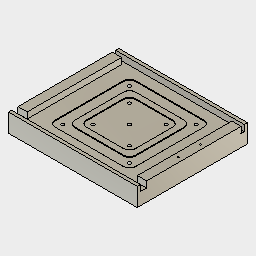
top (Autodesk Fusion 360 design; units mm, degrees)
Autodesk Fusion 360 part; units mm, degrees
note: some values were not read from the file. Chosen so that the rebuilt part matches the saved one: which bodies a step acts on; which face or edge a step refers to. Set by a fixed rule: which sketch regions a step uses.
box "BoxPrimitive1" add length 114.3 width 133.35 height 19.05 placed x (0, 1, 0) y (-1, 0, 0) z (0, 0, 1) at (133.35, 0, 0) makes body 1 in component "Fillet"
fillet "Fillet1" radius 12.7 2 edges at (66.675, 0, 19.05) (66.675, 114.3, 19.05) on bodies 1 in component "Fillet"
box "BoxPrimitive1'" add length 114.3 width 133.35 height 19.05 placed x (0, 1, 0) y (-1, 0, 0) z (0, 0, 1) at (133.35, 0, 0) separate body makes body 2 in component "Inside"
sketch "Sketch2" plane through (0, 0, 19.05) normal (0, 0, 1) x (-1, 0, 0) in component "Inside"
  line L0 (-133.35, -114.3) -> (0, -114.3)
  line L1 (0, -114.3) -> (0, 0)
  line L2 (0, 0) -> (-133.35, 0)
  line L3 (-133.35, 0) -> (-133.35, -114.3)
  line L4 (0, -3.302) -> (-133.35, -3.302)
  line L5 (-133.35, -3.302) -> (-133.35, -9.779)
  line L6 (0, -9.779) -> (0, -3.302)
  line L7 (0, -110.998) -> (-133.35, -110.998)
  line L8 (-133.35, -110.998) -> (-133.35, -107.696)
  line L9 (0, -107.696) -> (0, -110.998)
  line L10 (-123.825, -107.696) -> (-123.825, -9.779)
  line L11 (-9.525, -107.696) -> (-9.525, -9.779)
  line L12 (-133.35, -107.696) -> (-123.825, -107.696)
  line L13 (-9.525, -107.696) -> (0, -107.696)
  line L14 (-133.35, -9.779) -> (-123.825, -9.779)
  line L15 (-9.525, -9.779) -> (0, -9.779)
extrude "Extrude1" cut sketch "Sketch2" against normal blind 6.35 contours L1 L3 L4 L5 L6 L7 L8 L9 L10 L11 L12 L13 L14 L15 bodies 2 in component "Inside"
box "BoxPrimitive1''" add length 50.8 width 50.8 height 0.8128 placed x (0, 1, 0) y (-1, 0, 0) z (0, 0, 1) at (50.8, 0, 0) separate body makes body 3 in component "Copper Touch Pad"
sketch "Sketch2 (2)" plane through (0, 0, 0.8128) normal (0, 0, 1) x (-1, 0, 0) in component "Copper Touch Pad"
  line L0 (-50.8, -50.8) -> (0, -50.8)
  line L1 (0, -50.8) -> (0, 0)
  line L2 (0, 0) -> (-50.8, 0)
  line L3 (-50.8, 0) -> (-50.8, -50.8)
  line L4 (-44.45, 0) -> (-6.35, 0)
  line L5 (0, -6.35) -> (0, -44.45)
  line L6 (-6.35, -50.8) -> (-44.45, -50.8)
  line L7 (-50.8, -44.45) -> (-50.8, -6.35)
  arc A0 (-6.35, -50.8) -> (0, -44.45) centre (-6.35, -44.45) ccw
  arc A1 (-50.8, -44.45) -> (-44.45, -50.8) centre (-44.45, -44.45) ccw
  arc A2 (-44.45, 0) -> (-50.8, -6.35) centre (-44.45, -6.35) ccw
  arc A3 (0, -6.35) -> (-6.35, 0) centre (-6.35, -6.35) ccw
  circle A4 centre (-6.35, -44.45) radius 2.413
  circle A5 centre (-44.45, -44.45) radius 2.413
  circle A6 centre (-6.35, -6.35) radius 2.413
  circle A7 centre (-44.45, -6.35) radius 2.413
  circle A8 centre (-25.4, -25.4) radius 2.413
  point P0 (-25.4, -25.4)
  point P1 (-25.4, -25.4)
  dimension "d116" = 6.35
  dimension "d117" = 4.826
  dimension "d118" = 4.826
  dimension "d119" = 4.826
  dimension "d120" = 4.826
  measures "d116" radius of A0
  measures "d117" diameter of A5
  measures "d118" diameter of A6
  measures "d119" diameter of A7
  measures "d120" diameter of A8
extrude "Extrude1'" cut sketch "Sketch2 (2)" against normal blind 0.8128 contours L0 L3 A1 | L0 L1 A0 | L2 L3 A2 | L1 L2 A3 bodies 3 in component "Copper Touch Pad"
extrude "Extrude2" cut sketch "Sketch2 (2)" against normal blind 0.8128 contours A4 | A5 | A6 | A7 | A8 bodies 3 in component "Copper Touch Pad"
box "BoxPrimitive2" add length 79.4258 width 131.7498 height 19.558 placed x (0, 1, 0) y (-1, 0, 0) z (0, 0, 1) at (131.7498, 0, 0) separate body makes body 4 in component "Touch Test Block"
sketch "Sketch4" plane through (0, 0, 19.558) normal (0, 0, 1) x (-1, 0, 0) in component "Touch Test Block"
  line L0 (-131.7498, -79.4258) -> (0, -79.4258)
  line L1 (0, -79.4258) -> (0, 0)
  line L2 (0, 0) -> (-131.7498, 0)
  line L3 (-131.7498, 0) -> (-131.7498, -79.4258)
  line L4 (-84.9249, -14.3129) -> (-46.8249, -14.3129)
  line L5 (-40.4749, -20.6629) -> (-40.4749, -58.7629)
  line L6 (-46.8249, -65.1129) -> (-84.9249, -65.1129)
  line L7 (-91.2749, -58.7629) -> (-91.2749, -20.6629)
  line L8 (-125.5649, -5.4229) -> (-6.1849, -5.4229)
  line L9 (-6.1849, -5.4229) -> (-6.1849, -74.0029)
  line L10 (-6.1849, -74.0029) -> (-125.5649, -74.0029)
  line L11 (-131.7498, -37.1729) -> (-125.5651, -37.1729)
  line L12 (-125.5651, -42.2529) -> (-131.7498, -42.2529)
  line L13 (-131.7498, -42.2529) -> (-131.7498, -37.1729)
  arc A0 (-46.8249, -65.1129) -> (-40.4749, -58.7629) centre (-46.8249, -58.7629) ccw
  arc A1 (-91.2749, -58.7629) -> (-84.9249, -65.1129) centre (-84.9249, -58.7629) ccw
  arc A2 (-84.9249, -14.3129) -> (-91.2749, -20.6629) centre (-84.9249, -20.6629) ccw
  arc A3 (-40.4749, -20.6629) -> (-46.8249, -14.3129) centre (-46.8249, -20.6629) ccw
  circle A4 centre (-46.8249, -58.7629) radius 1.651
  circle A5 centre (-84.9249, -58.7629) radius 1.651
  circle A6 centre (-65.8749, -39.7129) radius 1.651
  circle A7 centre (-46.8249, -20.6629) radius 1.651
  circle A8 centre (-84.9249, -20.6629) radius 1.651
  line L14 (-125.5649, -74.0029) -> (-125.5651, -42.2529)
  line L15 (-125.5651, -37.1729) -> (-125.5649, -5.4229)
  point P0 (-65.8749, -39.7129)
  point P1 (-65.8749, -39.7129)
  point P2 (-65.8749, -39.7129)
  point P3 (-128.6574, -39.7129)
  point P4 (-128.6574, -39.7129)
  dimension "d149" = 6.35
  measures "d149" radius of A0
extrude "Extrude3" cut sketch "Sketch4" against normal blind 6.35 contours L3 L8 L9 L10 L11 L12 L13 L14 L15 bodies 4 in component "Touch Test Block"
extrude "Extrude4" cut sketch "Sketch4" against normal blind 7.1628 contours L4 L5 L6 L7 A0 A1 A2 A3 bodies 4 in component "Touch Test Block"
extrude "Extrude5" cut sketch "Sketch4" against normal blind 15.875 contours A4 | A5 | A6 | A7 | A8 bodies 4 in component "Touch Test Block"
box "BoxPrimitive1'''" add length 114.3 width 133.35 height 19.05 placed x (0, 1, 0) y (-1, 0, 0) z (0, 0, 1) at (133.35, 0, 0) separate body makes body 5 in component "Inside w/ Touch and Ring"
extrude "Extrude1''" cut sketch "Sketch2" against normal blind 6.35 contours L1 L3 L4 L5 L6 L7 L8 L9 L10 L11 L12 L13 L14 L15 bodies 5 in component "Inside w/ Touch and Ring"
sketch "Sketch2 (3)" plane through (0, 0, 12.7) normal (0, 0, 1) x (-1, 0, 0) in component "Inside w/ Touch and Ring"
  line L0 (-9.525, -107.696) -> (-9.525, -9.779)
  line L1 (-9.525, -9.779) -> (0, -9.779)
  line L2 (0, -9.779) -> (0, -3.302)
  line L3 (0, -3.302) -> (-133.35, -3.302)
  line L4 (-133.35, -3.302) -> (-133.35, -9.779)
  line L5 (-133.35, -9.779) -> (-123.825, -9.779)
  line L6 (-123.825, -9.779) -> (-123.825, -107.696)
  line L7 (-123.825, -107.696) -> (-133.35, -107.696)
  line L8 (-133.35, -107.696) -> (-133.35, -110.998)
  line L9 (-133.35, -110.998) -> (0, -110.998)
  line L10 (0, -110.998) -> (0, -107.696)
  line L11 (0, -107.696) -> (-9.525, -107.696)
  circle A0 centre (-47.625, -77.7875) radius 1.651
  circle A1 centre (-85.725, -77.7875) radius 1.651
  circle A2 centre (-85.725, -39.6875) radius 1.651
  circle A3 centre (-47.625, -39.6875) radius 1.651
  line L12 (-47.498, -33.2105) -> (-85.852, -33.2105)
  line L13 (-92.202, -39.5605) -> (-92.202, -77.9145)
  line L14 (-85.852, -84.2645) -> (-47.498, -84.2645)
  line L15 (-41.148, -77.9145) -> (-41.148, -39.5605)
  arc A4 (-47.498, -84.2645) -> (-41.148, -77.9145) centre (-47.498, -77.9145) ccw
  arc A5 (-92.202, -77.9145) -> (-85.852, -84.2645) centre (-85.852, -77.9145) ccw
  arc A6 (-85.852, -33.2105) -> (-92.202, -39.5605) centre (-85.852, -39.5605) ccw
  arc A7 (-41.148, -39.5605) -> (-47.498, -33.2105) centre (-47.498, -39.5605) ccw
  circle A8 centre (-66.675, -58.7375) radius 1.651
  point P0 (-66.675, -58.7375)
  point P1 (-66.675, -58.7375)
  point P2 (-66.675, -58.7375)
  dimension "d171" = 6.35
  measures "d171" radius of A4
extrude "Extrude2'" cut sketch "Sketch2 (3)" against normal blind 0.8128 contours L12 L13 L14 L15 A4 A5 A6 A7 bodies 5 in component "Inside w/ Touch and Ring"
extrude "Extrude3'" cut sketch "Sketch2 (3)" against normal blind 9.779 contours A0 | A1 | A2 | A3 | A8 bodies 5 in component "Inside w/ Touch and Ring"
box "BoxPrimitive1''''" add length 88.9 width 88.9 height 0.8128 placed x (0, 1, 0) y (-1, 0, 0) z (0, 0, 1) at (88.9, 0, 0) separate body makes body 6 in component "Copper Touch Pad w/ Ring"
sketch "Sketch2 (4)" plane through (0, 0, 0.8128) normal (0, 0, 1) x (-1, 0, 0) in component "Copper Touch Pad w/ Ring"
  line L0 (-88.9, -88.9) -> (0, -88.9)
  line L1 (0, -88.9) -> (0, 0)
  line L2 (0, 0) -> (-88.9, 0)
  line L3 (-88.9, 0) -> (-88.9, -88.9)
  line L4 (-69.85, -12.7) -> (-19.05, -12.7)
  line L5 (-12.7, -19.05) -> (-12.7, -69.85)
  line L6 (-19.05, -76.2) -> (-69.85, -76.2)
  line L7 (-76.2, -69.85) -> (-76.2, -19.05)
  arc A0 (-19.05, -76.2) -> (-12.7, -69.85) centre (-19.05, -69.85) ccw
  arc A1 (-76.2, -69.85) -> (-69.85, -76.2) centre (-69.85, -69.85) ccw
  arc A2 (-69.85, -12.7) -> (-76.2, -19.05) centre (-69.85, -19.05) ccw
  arc A3 (-12.7, -19.05) -> (-19.05, -12.7) centre (-19.05, -19.05) ccw
  point P0 (-44.45, -44.45)
  point P1 (-44.45, -44.45)
  dimension "d183" = 6.35
  dimension "d184" = 6.35
  measures "d183" radius of A0
  measures "d184" radius of A1
extrude "Extrude1'''" cut sketch "Sketch2 (4)" against normal blind 0.8128 contours L4 L5 L6 L7 A0 A1 A2 A3 bodies 6 in component "Copper Touch Pad w/ Ring"
fillet "Fillet1'" radius 6.35 1 edges at (88.9, 0, 0.4064) on bodies 6 in component "Copper Touch Pad w/ Ring"
fillet "Fillet2" radius 6.35 1 edges at (88.9, 88.9, 0.4064) on bodies 6 in component "Copper Touch Pad w/ Ring"
fillet "Fillet3" radius 6.35 1 edges at (0, 88.9, 0.4064) on bodies 6 in component "Copper Touch Pad w/ Ring"
fillet "Fillet4" radius 6.35 1 edges at (0, 0, 0.4064) on bodies 6 in component "Copper Touch Pad w/ Ring"
sketch "Sketch3" plane through (0, 0, 0.8128) normal (0, 0, 1) x (-1, 0, 0) in component "Copper Touch Pad w/ Ring"
  line L0 (-6.35, 0) -> (-82.55, 0)
  circle A0 centre (-81.28, -7.62) radius 2.413
  circle A1 centre (-7.62, -7.62) radius 2.413
  circle A2 centre (-7.62, -81.28) radius 2.413
  circle A3 centre (-81.28, -81.28) radius 2.413
  dimension "d191" = 4.826
  dimension "d192" = 4.826
  dimension "d193" = 4.826
  dimension "d194" = 4.826
  measures "d191" diameter of A0
  measures "d192" diameter of A1
  measures "d193" diameter of A2
  measures "d194" diameter of A3
extrude "Extrude2''" cut sketch "Sketch3" against normal blind 0.8128 bodies 6 in component "Copper Touch Pad w/ Ring"
sketch "Sketch3 (2)" plane through (0, 0, 12.7) normal (0, 0, 1) x (-1, 0, 0) in component "Inside w/ Touch and Ring"
  line L0 (-9.525, -107.696) -> (-9.525, -9.779)
  line L1 (-9.525, -9.779) -> (0, -9.779)
  line L2 (0, -9.779) -> (0, -3.302)
  line L3 (0, -3.302) -> (-133.35, -3.302)
  line L4 (-133.35, -3.302) -> (-133.35, -9.779)
  line L5 (-133.35, -9.779) -> (-123.825, -9.779)
  line L6 (-123.825, -9.779) -> (-123.825, -107.696)
  line L7 (-123.825, -107.696) -> (-133.35, -107.696)
  line L8 (-133.35, -107.696) -> (-133.35, -110.998)
  line L9 (-133.35, -110.998) -> (0, -110.998)
  line L10 (0, -110.998) -> (0, -107.696)
  line L11 (0, -107.696) -> (-9.525, -107.696)
  line L12 (-85.852, -33.2105) -> (-47.498, -33.2105)
  arc A0 (-41.148, -39.5605) -> (-47.498, -33.2105) centre (-47.498, -39.5605) ccw
  line L13 (-41.148, -39.5605) -> (-41.148, -77.9145)
  arc A1 (-47.498, -84.2645) -> (-41.148, -77.9145) centre (-47.498, -77.9145) ccw
  line L14 (-47.498, -84.2645) -> (-85.852, -84.2645)
  arc A2 (-92.202, -77.9145) -> (-85.852, -84.2645) centre (-85.852, -77.9145) ccw
  line L15 (-92.202, -77.9145) -> (-92.202, -39.5605)
  arc A3 (-85.852, -33.2105) -> (-92.202, -39.5605) centre (-85.852, -39.5605) ccw
  line L16 (-97.79, -27.6225) -> (-41.91, -27.6225)
  line L17 (-35.56, -33.9725) -> (-35.56, -89.8525)
  line L18 (-35.56, -89.8525) -> (-97.79, -89.8525)
  line L19 (-97.79, -89.8525) -> (-97.79, -27.6225)
  line L20 (-97.79, -27.6225) -> (-35.56, -89.8525) construction
  line L21 (-35.56, -27.6225) -> (-97.79, -89.8525) construction
  arc A4 (-35.56, -33.9725) -> (-41.91, -27.6225) centre (-41.91, -33.9725) ccw
  line L22 (-106.68, -18.7325) -> (-33.02, -18.7325)
  line L23 (-26.67, -25.0825) -> (-26.67, -98.7425)
  line L24 (-26.67, -98.7425) -> (-106.68, -98.7425)
  line L25 (-106.68, -98.7425) -> (-106.68, -18.7325)
  line L26 (-106.68, -18.7325) -> (-26.67, -98.7425) construction
  arc A5 (-26.67, -25.0825) -> (-33.02, -18.7325) centre (-33.02, -25.0825) ccw
  circle A6 centre (-33.02, -25.0825) radius 1.651
  point P0 (-66.675, -58.7375)
  point P1 (-66.675, -58.7375)
  point P2 (-66.675, -58.7375)
  dimension "d202" = 80.01
  dimension "d204" = 6.35
  measures "d202" distance of L23.end L24.end
  measures "d204" radius of A5
box "BoxPrimitive2'" add length 82.55 width 82.55 height 0.8128 placed x (0, 1, 0) y (-1, 0, 0) z (0, 0, 1) at (82.55, 0, 0) separate body makes body 7 in component "Copper Touch Pad w/ Ring"
sketch "Sketch5" plane through (0, 0, 0.8128) normal (0, 0, 1) x (-1, 0, 0) in component "Copper Touch Pad w/ Ring"
  line L0 (-82.55, -82.55) -> (0, -82.55)
  line L1 (0, -82.55) -> (0, 0)
  line L2 (0, 0) -> (-82.55, 0)
  line L3 (-82.55, 0) -> (-82.55, -82.55)
  line L4 (0, -82.55) -> (-82.55, 0)
  line L5 (0, 0) -> (-82.55, -82.55)
  line L6 (-66.675, -9.525) -> (-15.875, -9.525)
  line L7 (-9.525, -15.875) -> (-9.525, -66.675)
  line L8 (-15.875, -73.025) -> (-66.675, -73.025)
  line L9 (-73.025, -66.675) -> (-73.025, -15.875)
  line L10 (-73.025, -9.525) -> (-9.525, -73.025) construction
  line L11 (-9.525, -9.525) -> (-73.025, -73.025) construction
  arc A0 (-73.025, -66.675) -> (-66.675, -73.025) centre (-66.675, -66.675) ccw
  line L12 (-76.2, 0) -> (-6.35, 0)
  line L13 (0, -6.35) -> (0, -76.2)
  line L14 (-6.35, -82.55) -> (-76.2, -82.55)
  line L15 (-82.55, -76.2) -> (-82.55, -6.35)
  line L16 (-82.55, 0) -> (0, -82.55) construction
  line L17 (0, 0) -> (-82.55, -82.55) construction
  arc A1 (-82.55, -76.2) -> (-76.2, -82.55) centre (-76.2, -76.2) ccw
  line L18 (-71.1651, -71.1651) -> (-75.9247, -75.9247)
  circle A2 centre (-75.9247, -75.9247) radius 2.413
  arc A3 (-6.35, -82.55) -> (0, -76.2) centre (-6.35, -76.2) ccw
  arc A4 (-15.875, -73.025) -> (-9.525, -66.675) centre (-15.875, -66.675) ccw
  line L19 (-11.3849, -71.1651) -> (-6.6253, -75.9247)
  circle A5 centre (-6.6253, -75.9247) radius 2.413
  arc A6 (0, -6.35) -> (-6.35, 0) centre (-6.35, -6.35) ccw
  arc A7 (-9.525, -15.875) -> (-15.875, -9.525) centre (-15.875, -15.875) ccw
  line L20 (-11.3849, -11.3849) -> (-6.6253, -6.6253)
  circle A8 centre (-6.6253, -6.6253) radius 2.413
  arc A9 (-76.2, 0) -> (-82.55, -6.35) centre (-76.2, -6.35) ccw
  arc A10 (-66.675, -9.525) -> (-73.025, -15.875) centre (-66.675, -15.875) ccw
  line L21 (-71.1651, -11.3849) -> (-75.9247, -6.6253)
  circle A11 centre (-75.9247, -6.6253) radius 2.413
  line L22 (-60.325, -15.875) -> (-22.225, -15.875)
  line L23 (-15.875, -22.225) -> (-15.875, -60.325)
  line L24 (-22.225, -66.675) -> (-60.325, -66.675)
  line L25 (-66.675, -60.325) -> (-66.675, -22.225)
  line L26 (-66.675, -15.875) -> (-15.875, -66.675) construction
  line L27 (-15.875, -15.875) -> (-66.675, -66.675) construction
  arc A12 (-22.225, -66.675) -> (-15.875, -60.325) centre (-22.225, -60.325) ccw
  arc A13 (-66.675, -60.325) -> (-60.325, -66.675) centre (-60.325, -60.325) ccw
  arc A14 (-60.325, -15.875) -> (-66.675, -22.225) centre (-60.325, -22.225) ccw
  arc A15 (-15.875, -22.225) -> (-22.225, -15.875) centre (-22.225, -22.225) ccw
  circle A16 centre (-22.225, -60.325) radius 2.413
  circle A17 centre (-60.325, -60.325) radius 2.413
  circle A18 centre (-60.325, -22.225) radius 2.413
  circle A19 centre (-22.225, -22.225) radius 2.413
  circle A20 centre (-41.275, -41.275) radius 2.413
  point P0 (-41.275, -41.275)
  point P1 (-41.275, -41.275)
  point P2 (-80.6901, -80.6901)
  point P3 (-71.1651, -71.1651)
  point P4 (-41.275, -41.275)
  dimension "d213" = 6.35
  dimension "d214" = 4.826
  dimension "d215" = 6.35
  dimension "d216" = 6.35
  dimension "d217" = 6.731
  dimension "d218" = 4.826
  dimension "d219" = 6.35
  dimension "d220" = 6.35
  dimension "d221" = 6.731
  dimension "d222" = 4.826
  dimension "d223" = 6.35
  dimension "d224" = 6.35
  dimension "d225" = 6.731
  dimension "d226" = 4.826
  dimension "d227" = 50.8
  dimension "d228" = 50.8
  dimension "d229" = 6.35
  dimension "d230" = 4.826
  dimension "d231" = 4.826
  dimension "d232" = 4.826
  dimension "d233" = 4.826
  dimension "d234" = 4.826
  measures "d213" radius of A1
  measures "d214" diameter of A2
  measures "d215" radius of A3
  measures "d216" radius of A4
  measures "d217" distance of L19.start L19.end
  measures "d218" diameter of A5
  measures "d219" radius of A6
  measures "d220" radius of A7
  measures "d221" distance of L20.start L20.end
  measures "d222" diameter of A8
  measures "d223" radius of A9
  measures "d224" radius of A10
  measures "d225" distance of L21.start L21.end
  measures "d226" diameter of A11
  measures "d227" distance of A4.centre A0.centre
  measures "d228" distance of A7.centre A4.centre
  measures "d229" radius of A12
  measures "d230" diameter of A16
  measures "d231" diameter of A17
  measures "d232" diameter of A18
  measures "d233" diameter of A19
  measures "d234" diameter of A20
extrude "Extrude3''" cut sketch "Sketch5" against normal blind 0.8128 contours L0 L5 A1 | L3 L5 A1 | L0 L4 A3 | L3 L4 A9 | L5 L18 A2 | L5 L18 A2 | L1 L4 A3 | L2 L4 A9 | L4 L19 A5 | L4 L19 A5 | L4 L21 A11 | L4 L21 A11 | L4 L5 L9 A0 A10 L25 A13 A14 | L4 L5 L8 A0 A4 L24 A12 A13 | L1 L5 A6 | L2 L5 A6 | L4 L5 L7 A4 A7 L23 A12 A15 | L4 L5 L6 A7 A10 L22 A14 A15 | L5 A17 | L5 A17 | L5 L20 A8 | L5 L20 A8 | L4 A16 | L4 A16 | L4 A18 | L4 A18 | L4 L5 A20 | L4 L5 A20 | L4 L5 A20 | L4 L5 A20 | L5 A19 | L5 A19 bodies 7 makes body 8 at (32.8083, 3.175, 0.8128) in component "Copper Touch Pad w/ Ring"
sketch "Sketch4 (2)" plane through (0, 0, 12.7) normal (0, 0, 1) x (-1, 0, 0) in component "Inside w/ Touch and Ring"
  line L0 (-9.525, -107.696) -> (-9.525, -9.779)
  line L1 (-9.525, -9.779) -> (0, -9.779)
  line L2 (0, -9.779) -> (0, -3.302)
  line L3 (0, -3.302) -> (-133.35, -3.302)
  line L4 (-133.35, -3.302) -> (-133.35, -9.779)
  line L5 (-133.35, -9.779) -> (-123.825, -9.779)
  line L6 (-123.825, -9.779) -> (-123.825, -107.696)
  line L7 (-123.825, -107.696) -> (-133.35, -107.696)
  line L8 (-133.35, -107.696) -> (-133.35, -110.998)
  line L9 (-133.35, -110.998) -> (0, -110.998)
  line L10 (0, -110.998) -> (0, -107.696)
  line L11 (0, -107.696) -> (-9.525, -107.696)
  line L12 (-85.852, -33.2105) -> (-47.498, -33.2105)
  arc A0 (-41.148, -39.5605) -> (-47.498, -33.2105) centre (-47.498, -39.5605) ccw
  line L13 (-41.148, -39.5605) -> (-41.148, -77.9145)
  arc A1 (-47.498, -84.2645) -> (-41.148, -77.9145) centre (-47.498, -77.9145) ccw
  line L14 (-47.498, -84.2645) -> (-85.852, -84.2645)
  arc A2 (-92.202, -77.9145) -> (-85.852, -84.2645) centre (-85.852, -77.9145) ccw
  line L15 (-92.202, -77.9145) -> (-92.202, -39.5605)
  arc A3 (-85.852, -33.2105) -> (-92.202, -39.5605) centre (-85.852, -39.5605) ccw
  line L16 (-47.4345, -84.3915) -> (-85.9155, -84.3915)
  line L17 (-91.821, -27.305) -> (-41.529, -27.305)
  line L18 (-101.9492, -17.0498) -> (-31.4008, -17.0498)
  line L19 (-85.9155, -33.0835) -> (-47.4345, -33.0835)
  arc A4 (-101.9492, -17.0498) -> (-108.3627, -23.4633) centre (-101.9492, -23.4632) ccw
  arc A5 (-91.821, -27.305) -> (-98.1075, -33.5915) centre (-91.821, -33.5915) ccw
  line L20 (-41.021, -39.497) -> (-41.021, -77.978)
  line L21 (-24.9872, -23.4633) -> (-24.9872, -94.0118)
  line L22 (-35.2425, -33.5915) -> (-35.2425, -83.8835)
  line L23 (-31.4008, -100.4253) -> (-101.9492, -100.4253)
  line L24 (-108.3628, -94.0118) -> (-108.3628, -23.4633)
  arc A6 (-41.021, -39.497) -> (-47.4345, -33.0835) centre (-47.4345, -39.497) ccw
  arc A7 (-85.9155, -33.0835) -> (-92.329, -39.497) centre (-85.9155, -39.497) ccw
  arc A8 (-92.329, -77.978) -> (-85.9155, -84.3915) centre (-85.9155, -77.978) ccw
  arc A9 (-47.4345, -84.3915) -> (-41.021, -77.978) centre (-47.4345, -77.978) ccw
  line L25 (-41.529, -90.17) -> (-91.821, -90.17)
  arc A10 (-41.529, -90.17) -> (-35.2425, -83.8835) centre (-41.529, -83.8835) ccw
  arc A11 (-31.4008, -100.4253) -> (-24.9872, -94.0118) centre (-31.4007, -94.0118) ccw
  line L26 (-98.1075, -83.8835) -> (-98.1075, -33.5915)
  line L27 (-92.329, -77.978) -> (-92.329, -39.497)
  arc A12 (-98.1075, -83.8835) -> (-91.821, -90.17) centre (-91.821, -83.8835) ccw
  arc A13 (-108.3628, -94.0118) -> (-101.9492, -100.4253) centre (-101.9492, -94.0118) ccw
  arc A14 (-35.2425, -33.5915) -> (-41.529, -27.305) centre (-41.529, -33.5915) ccw
  arc A15 (-24.9872, -23.4633) -> (-31.4008, -17.0498) centre (-31.4007, -23.4633) ccw
  circle A16 centre (-32.0253, -93.3872) radius 1.651
  circle A17 centre (-101.3247, -93.3872) radius 1.651
  circle A18 centre (-32.0253, -24.0878) radius 1.651
  circle A19 centre (-101.3247, -24.0878) radius 1.651
  circle A20 centre (-47.625, -77.7875) radius 1.651
  circle A21 centre (-66.675, -58.7375) radius 1.651
  circle A22 centre (-47.625, -39.6875) radius 1.651
  circle A23 centre (-85.725, -39.6875) radius 1.651
  circle A24 centre (-85.725, -77.7875) radius 1.651
  point P0 (-25.4, -17.4625)
  point P1 (-66.675, -58.7375)
  point P2 (-66.675, -58.7375)
  point P3 (-106.0901, -98.1526)
  point P4 (-96.5651, -88.6276)
  point P5 (-66.675, -58.7375)
  dimension "d269" = 3.302
  measures "d269" diameter of A22
extrude "Extrude4'" add 1 faces at (80.0076, 58.7375, 11.8872) along direction (0, 0, 1) blind 0.8128 on bodies 5 bodies 5 in component "Inside w/ Touch and Ring"
extrude "Extrude5'" add 5 faces at (67.1105, 59.7809, 2.921) (48.2808, 39.8898, 2.921) (48.5864, 78.1325, 2.921) (85.9261, 78.7774, 2.921) (86.1605, 40.7309, 2.921) along direction (0, 0, 1) blind 9.779 on bodies 5 bodies 5 in component "Inside w/ Touch and Ring"
extrude "Extrude6" cut sketch "Sketch4 (2)" against normal blind 9.779 contours A16 | A17 | A18 | A19 | A20 | A21 | A22 | A23 | A24 bodies 5 in component "Inside w/ Touch and Ring"
extrude "Extrude7" cut sketch "Sketch4 (2)" against normal blind 0.8128 contours L12 A0 L13 A1 L14 A2 L15 A3 | L18 A4 L21 L23 L24 A11 A13 A15 bodies 5 in component "Inside w/ Touch and Ring"
move_body "Move1" bodies 8 7 to x (1, 0, 0) y (0, 1, 0) z (0, 0, 1) at (2.54, 2.54, 0) in component "Copper Touch Pad w/ Ring"
sketch "Sketch5 (2)" plane through (0, 0, 19.05) normal (0, 0, 1) x (-1, 0, 0) in component "Inside w/ Touch and Ring"
  line L0 (-133.35, -107.696) -> (-123.825, -107.696)
  line L1 (-123.825, -107.696) -> (-123.825, -9.779)
  line L2 (-123.825, -9.779) -> (-133.35, -9.779)
  line L3 (-133.35, -9.779) -> (-133.35, -107.696)
  line L4 (-128.5875, -58.7375) -> (-128.5875, -70.2361)
  line L5 (-128.5875, -58.7375) -> (-128.5875, -47.2389)
  circle A0 centre (-128.5875, -70.2361) radius 0.8001
  circle A1 centre (-128.5875, -47.2389) radius 0.8001
  point P0 (-128.5875, -58.7375)
  dimension "d276" = 11.4986
  dimension "d277" = 11.4986
  dimension "d278" = 1.6002
  dimension "d279" = 1.6002
  measures "d276" distance of P0 L4.end
  measures "d277" distance of P0 L5.end
  measures "d278" diameter of A0
  measures "d279" diameter of A1
extrude "Extrude8" cut sketch "Sketch5 (2)" against normal blind 4.7625 contours A0 | A1 bodies 5 in component "Inside w/ Touch and Ring"
box "BoxPrimitive1'''''" add length 50.8 width 50.8 height 0.8128 placed x (0, 1, 0) y (-1, 0, 0) z (0, 0, 1) at (50.8, 0, 0) separate body makes body 9 in component "Small Copper Touch Pad w/ Ring"
sketch "Sketch2 (5)" plane through (0, 0, 0.8128) normal (0, 0, 1) x (-1, 0, 0) in component "Small Copper Touch Pad w/ Ring"
  line L0 (-50.8, -50.8) -> (0, -50.8)
  line L1 (0, -50.8) -> (0, 0)
  line L2 (0, 0) -> (-50.8, 0)
  line L3 (-50.8, 0) -> (-50.8, -50.8)
  line L4 (-31.75, -12.7) -> (-19.05, -12.7)
  line L5 (-12.7, -19.05) -> (-12.7, -31.75)
  line L6 (-19.05, -38.1) -> (-31.75, -38.1)
  line L7 (-38.1, -31.75) -> (-38.1, -19.05)
  line L8 (-36.83, -7.62) -> (-13.97, -7.62)
  line L9 (-7.62, -13.97) -> (-7.62, -36.83)
  line L10 (-13.97, -43.18) -> (-36.83, -43.18)
  line L11 (-43.18, -36.83) -> (-43.18, -13.97)
  line L12 (-44.45, 0) -> (-6.35, 0)
  line L13 (0, -6.35) -> (0, -44.45)
  line L14 (-6.35, -50.8) -> (-44.45, -50.8)
  line L15 (-50.8, -44.45) -> (-50.8, -6.35)
  arc A0 (-6.35, -50.8) -> (0, -44.45) centre (-6.35, -44.45) ccw
  arc A1 (-50.8, -44.45) -> (-44.45, -50.8) centre (-44.45, -44.45) ccw
  arc A2 (-44.45, 0) -> (-50.8, -6.35) centre (-44.45, -6.35) ccw
  arc A3 (0, -6.35) -> (-6.35, 0) centre (-6.35, -6.35) ccw
  arc A4 (-7.62, -13.97) -> (-13.97, -7.62) centre (-13.97, -13.97) ccw
  arc A5 (-36.83, -7.62) -> (-43.18, -13.97) centre (-36.83, -13.97) ccw
  arc A6 (-43.18, -36.83) -> (-36.83, -43.18) centre (-36.83, -36.83) ccw
  arc A7 (-13.97, -43.18) -> (-7.62, -36.83) centre (-13.97, -36.83) ccw
  arc A8 (-19.05, -38.1) -> (-12.7, -31.75) centre (-19.05, -31.75) ccw
  arc A9 (-38.1, -31.75) -> (-31.75, -38.1) centre (-31.75, -31.75) ccw
  arc A10 (-31.75, -12.7) -> (-38.1, -19.05) centre (-31.75, -19.05) ccw
  arc A11 (-12.7, -19.05) -> (-19.05, -12.7) centre (-19.05, -19.05) ccw
  circle A12 centre (-45.085, -45.085) radius 2.413
  circle A13 centre (-5.715, -45.085) radius 2.413
  circle A14 centre (-5.715, -5.715) radius 2.413
  circle A15 centre (-45.085, -5.715) radius 2.413
  circle A16 centre (-25.4, -25.4) radius 2.413
  point P0 (-25.4, -25.4)
  point P1 (-25.4, -25.4)
  point P2 (-25.4, -25.4)
  dimension "d289" = 6.35
  dimension "d290" = 4.826
  dimension "d291" = 4.826
  dimension "d292" = 4.826
  dimension "d293" = 4.826
  dimension "d294" = 4.826
  measures "d289" radius of A0
  measures "d290" diameter of A12
  measures "d291" diameter of A13
  measures "d292" diameter of A14
  measures "d293" diameter of A15
  measures "d294" diameter of A16
extrude "Extrude1''''" cut sketch "Sketch2 (5)" against normal blind 0.8128 contours L0 L3 A1 | L0 L1 A0 | L2 L3 A2 | L1 L2 A3 | L8 L9 L10 L11 A4 A5 A6 A7 | A12 | A13 | A14 | A15 | A16 bodies 9 makes body 10 at (25.3399, 16.1312, 0.8128) in component "Small Copper Touch Pad w/ Ring"
box "BoxPrimitive1''''''" add length 114.3 width 133.35 height 19.05 placed x (0, 1, 0) y (-1, 0, 0) z (0, 0, 1) at (133.35, 0, 0) separate body makes body 11 in component "Inside w/ Small Touch"
sketch "Sketch2 (6)" plane through (0, 0, 19.05) normal (0, 0, 1) x (-1, 0, 0) in component "Inside w/ Small Touch"
  line L0 (-133.35, -114.3) -> (0, -114.3)
  line L1 (0, -114.3) -> (0, 0)
  line L2 (0, 0) -> (-133.35, 0)
  line L3 (-133.35, 0) -> (-133.35, -114.3)
  line L4 (0, -3.302) -> (-133.35, -3.302)
  line L5 (-133.35, -3.302) -> (-133.35, -9.779)
  line L6 (0, -9.779) -> (0, -3.302)
  line L7 (0, -110.998) -> (-133.35, -110.998)
  line L8 (-133.35, -110.998) -> (-133.35, -107.696)
  line L9 (0, -107.696) -> (0, -110.998)
  line L10 (-123.825, -107.696) -> (-123.825, -9.779)
  line L11 (-9.525, -107.696) -> (-9.525, -9.779)
  line L12 (-133.35, -107.696) -> (-123.825, -107.696)
  line L13 (-9.525, -107.696) -> (0, -107.696)
  line L14 (-133.35, -9.779) -> (-123.825, -9.779)
  line L15 (-9.525, -9.779) -> (0, -9.779)
extrude "Extrude1'''''" cut sketch "Sketch2 (6)" against normal blind 6.35 contours L1 L3 L4 L5 L6 L7 L8 L9 L10 L11 L12 L13 L14 L15 bodies 11 in component "Inside w/ Small Touch"
sketch "Sketch3 (3)" plane through (0, 0, 12.7) normal (0, 0, 1) x (-1, 0, 0) in component "Inside w/ Small Touch"
  line L0 (-9.525, -107.696) -> (-9.525, -9.779)
  line L1 (-9.525, -9.779) -> (0, -9.779)
  line L2 (0, -9.779) -> (0, -3.302)
  line L3 (0, -3.302) -> (-133.35, -3.302)
  line L4 (-133.35, -3.302) -> (-133.35, -9.779)
  line L5 (-133.35, -9.779) -> (-123.825, -9.779)
  line L6 (-123.825, -9.779) -> (-123.825, -107.696)
  line L7 (-123.825, -107.696) -> (-133.35, -107.696)
  line L8 (-133.35, -107.696) -> (-133.35, -110.998)
  line L9 (-133.35, -110.998) -> (0, -110.998)
  line L10 (0, -110.998) -> (0, -107.696)
  line L11 (0, -107.696) -> (-9.525, -107.696)
  line L12 (-53.7197, -52.2599) -> (-53.7197, -65.0869)
  arc A0 (-60.1332, -71.5004) -> (-53.7197, -65.0869) centre (-60.1332, -65.0869) ccw
  line L13 (-92.2007, -77.9139) -> (-92.2007, -39.4329)
  line L14 (-60.1332, -71.5004) -> (-72.9602, -71.5004)
  arc A1 (-40.8927, -39.4329) -> (-47.3062, -33.0194) centre (-47.3062, -39.4329) ccw
  line L15 (-79.3737, -65.0869) -> (-79.3737, -52.2599)
  line L16 (-48.9471, -47.3589) -> (-48.9471, -69.9903)
  line L17 (-47.3062, -84.3274) -> (-85.7872, -84.3274)
  arc A2 (-72.9602, -45.8464) -> (-79.3737, -52.2599) centre (-72.9602, -52.2599) ccw
  arc A3 (-55.2336, -76.2768) -> (-48.9471, -69.9903) centre (-55.2336, -69.9903) ccw
  line L18 (-72.9602, -45.8464) -> (-60.1332, -45.8464)
  arc A4 (-47.3062, -84.3274) -> (-40.8927, -77.9139) centre (-47.3062, -77.9139) ccw
  arc A5 (-92.2007, -77.9139) -> (-85.7872, -84.3274) centre (-85.7872, -77.9139) ccw
  arc A6 (-84.1515, -69.9903) -> (-77.865, -76.2768) centre (-77.865, -69.9903) ccw
  line L19 (-84.1515, -69.9903) -> (-84.1515, -47.3589)
  arc A7 (-48.9471, -47.3589) -> (-55.2336, -41.0724) centre (-55.2336, -47.3589) ccw
  arc A8 (-53.7197, -52.2599) -> (-60.1332, -45.8464) centre (-60.1332, -52.2599) ccw
  arc A9 (-77.865, -41.0724) -> (-84.1515, -47.3589) centre (-77.865, -47.3589) ccw
  line L20 (-85.7872, -33.0194) -> (-47.3062, -33.0194)
  line L21 (-77.865, -41.0724) -> (-55.2336, -41.0724)
  line L22 (-55.2336, -76.2768) -> (-77.865, -76.2768)
  arc A10 (-79.3737, -65.0869) -> (-72.9602, -71.5004) centre (-72.9602, -65.0869) ccw
  arc A11 (-85.7872, -33.0194) -> (-92.2007, -39.4329) centre (-85.7872, -39.4329) ccw
  line L23 (-40.8927, -39.4329) -> (-40.8927, -77.9139)
  circle A12 centre (-46.863, -78.359) radius 1.651
  circle A13 centre (-86.233, -78.359) radius 1.651
  circle A14 centre (-66.675, -58.7375) radius 1.651
  circle A15 centre (-46.863, -38.989) radius 1.651
  circle A16 centre (-86.233, -38.989) radius 1.651
  point P0 (-66.675, -58.7375)
  point P1 (-66.675, -58.7375)
  point P2 (-66.675, -58.7375)
  point P3 (-66.675, -58.7375)
  point P4 (-41.148, -33.274)
  dimension "d303" = 3.302
  dimension "d304" = 3.302
  dimension "d305" = 3.302
  dimension "d306" = 3.302
  dimension "d307" = 3.302
  measures "d303" diameter of A12
  measures "d304" diameter of A13
  measures "d305" diameter of A14
  measures "d306" diameter of A15
  measures "d307" diameter of A16
extrude "Extrude2'''" cut sketch "Sketch3 (3)" against normal blind 9.525 contours A12 | A13 | A14 | A15 | A16 bodies 11 in component "Inside w/ Small Touch"
extrude "Extrude3'''" cut sketch "Sketch3 (3)" against normal blind 0.8128 contours L12 A0 L14 L15 A2 L18 A8 A10 | L13 A1 L17 A4 A5 L20 A11 L23 bodies 11 in component "Inside w/ Small Touch"
sketch "Sketch4 (3)" plane through (0, 0, 19.05) normal (0, 0, 1) x (-1, 0, 0) in component "Inside w/ Small Touch"
  line L0 (-133.35, -107.696) -> (-123.825, -107.696)
  line L1 (-123.825, -107.696) -> (-123.825, -9.779)
  line L2 (-123.825, -9.779) -> (-133.35, -9.779)
  line L3 (-133.35, -9.779) -> (-133.35, -107.696)
  line L4 (-133.35, -9.779) -> (-133.35, -107.696)
  line L5 (-133.35, -9.779) -> (-133.35, -107.696)
  line L6 (-133.35, -107.696) -> (-123.825, -107.696)
  line L7 (-123.825, -9.779) -> (-133.35, -9.779)
  line L8 (-123.825, -9.779) -> (-133.35, -9.779)
  line L9 (-123.825, -107.696) -> (-123.825, -9.779)
  line L10 (-133.35, -107.696) -> (-123.825, -107.696)
  line L11 (-123.825, -107.696) -> (-123.825, -9.779)
  circle A0 centre (-128.5875, -70.2361) radius 0.8001
  circle A1 centre (-128.5875, -47.2389) radius 0.8001
  circle A2 centre (-128.5875, -70.2361) radius 0.8001
  circle A3 centre (-128.5875, -47.2389) radius 0.8001
  line L12 (-128.5875, -58.7375) -> (-128.5875, -70.2361)
  line L13 (-128.5875, -58.7375) -> (-128.5875, -70.2361)
  line L14 (-128.5875, -58.7375) -> (-128.5875, -47.2389)
  line L15 (-128.5875, -58.7375) -> (-128.5875, -47.2389)
  point P0 (-128.5875, -58.7375)
  dimension "d312" = 11.4986
  dimension "d313" = 11.4986
  dimension "d314" = 1.6002
  dimension "d315" = 1.6002
  measures "d312" distance of P0 A0.centre
  measures "d313" distance of P0 A1.centre
  measures "d314" diameter of A0
  measures "d315" diameter of A1
extrude "Extrude4''" cut sketch "Sketch4 (3)" against normal blind 4.7625 contours A0 A2 | A1 A3 bodies 11 in component "Inside w/ Small Touch"
box "BoxPrimitive1'''''''" add length 76.2 width 76.2 height 0.8128 placed x (0, 1, 0) y (-1, 0, 0) z (0, 0, 1) at (76.2, 0, 0) separate body makes body 12 in component "Circular Touch"
sketch "Sketch2 (7)" plane through (0, 0, 0.8128) normal (0, 0, 1) x (-1, 0, 0) in component "Circular Touch"
  line L0 (-76.2, -76.2) -> (0, -76.2)
  line L1 (0, -76.2) -> (0, 0)
  line L2 (0, 0) -> (-76.2, 0)
  line L3 (-76.2, 0) -> (-76.2, -76.2)
  circle A0 centre (-38.1, -38.1) radius 38.1
  circle A1 centre (-38.1, -38.1) radius 25.4
  circle A2 centre (-38.1, -38.1) radius 29.21
  circle A3 centre (-71.755, -38.1) radius 2.413
  circle A4 centre (-38.1, -71.755) radius 2.413
  circle A5 centre (-4.445, -38.1) radius 2.413
  circle A6 centre (-38.1, -4.445) radius 2.413
  circle A7 centre (-38.1, -38.1) radius 2.413
  point P0 (-38.1, -38.1)
extrude "Extrude1''''''" cut sketch "Sketch2 (7)" against normal blind 0.8128 contours L0 L3 A0 | L0 L1 A0 | L2 L3 A0 | L1 L2 A0 | A2 | A3 | A4 | A5 | A6 | A7 bodies 12 makes body 13 at (20.4659, 39.4818, 0.8128) in component "Circular Touch"
box "BoxPrimitive1''''''''" add length 50.8 width 50.8 height 0.8128 placed x (0, 1, 0) y (-1, 0, 0) z (0, 0, 1) at (50.8, 0, 0) separate body makes body 14 in component "Small Circular Touch"
sketch "Sketch2 (8)" plane through (0, 0, 0.8128) normal (0, 0, 1) x (-1, 0, 0) in component "Small Circular Touch"
  line L0 (-50.8, -50.8) -> (0, -50.8)
  line L1 (0, -50.8) -> (0, 0)
  line L2 (0, 0) -> (-50.8, 0)
  line L3 (-50.8, 0) -> (-50.8, -50.8)
  circle A0 centre (-25.4, -25.4) radius 25.4
  circle A1 centre (-25.4, -25.4) radius 17.78
  circle A2 centre (-46.99, -25.4) radius 2.413
  circle A3 centre (-3.81, -25.4) radius 2.413
  circle A4 centre (-25.4, -25.4) radius 16.129
  circle A5 centre (-25.4, -25.4) radius 2.413
  point P0 (-25.4, -25.4)
extrude "Extrude1'''''''" cut sketch "Sketch2 (8)" against normal blind 0.8128 contours L0 L3 A0 | L0 L1 A0 | L2 L3 A0 | L1 L2 A0 | A1 | A2 | A3 | A5 bodies 14 makes body 15 at (13.912, 26.3212, 0.8128) in component "Small Circular Touch"
extrude "Extrude9" add 1 faces at (32.4911, 93.5494, 2.921) along direction (0, 0, 1) blind 3.175 on bodies 5 bodies 5 in component "Inside w/ Touch and Ring"
extrude "Extrude10" add 1 faces at (32.4911, 93.5494, 6.096) along direction (0, 0, 1) blind 0.254 on bodies 5 bodies 5 in component "Inside w/ Touch and Ring"
extrude "Extrude11" add 1 faces at (48.2733, 78.1618, 2.921) along direction (0, 0, 1) blind 3.429 on bodies 5 bodies 5 in component "Inside w/ Touch and Ring"
extrude "Extrude12" add 5 faces at (31.5324, 23.3215, 2.921) (48.2808, 39.8898, 2.921) (67.1105, 59.7809, 2.921) (86.0681, 78.6953, 2.921) (101.6678, 94.295, 2.921) along direction (0, 0, 1) blind 3.429 on bodies 5 bodies 5 in component "Inside w/ Touch and Ring"
extrude "Extrude13" add 2 faces at (86.1605, 40.7309, 2.921) (101.6678, 24.9957, 2.921) along direction (0, 0, 1) blind 3.429 on bodies 5 bodies 5 in component "Inside w/ Touch and Ring"
extrude "Extrude5''" add 5 faces at (47.5113, 78.7333, 3.175) (86.4341, 79.3489, 3.175) (67.1105, 59.7809, 3.175) (47.5188, 39.1913, 3.175) (86.6685, 40.0324, 3.175) along direction (0, 0, 1) blind 3.429 on bodies 11 bodies 11 in component "Inside w/ Small Touch"
extrude "Extrude6'" cut 5 faces at (47.5113, 78.7333, 6.604) (86.4341, 79.3489, 6.604) (67.1105, 59.7809, 6.604) (47.5188, 39.1913, 6.604) (86.6685, 40.0324, 6.604) along direction (0, 0, -1) blind 0.254 on bodies 11 bodies 11 in component "Inside w/ Small Touch"
box "BoxPrimitive1'''''''''" add length 114.3 width 133.35 height 22.098 placed x (0, 1, 0) y (-1, 0, 0) z (0, 0, 1) at (133.35, 0, 0) separate body makes body 16 in component "Face"
box "BoxPrimitive2''" add length 114.3 width 133.35 height 20.066 placed x (0, 1, 0) y (-1, 0, 0) z (0, 0, 1) at (133.35, 0, 0) separate body makes body 17 in component "Face"
box "BoxPrimitive3" add length 114.3 width 133.35 height 19.05 placed x (0, 1, 0) y (-1, 0, 0) z (0, 0, 1) at (133.35, 0, 0) separate body makes body 18 in component "Face"
component "Fillet" placed x (1, 0, 0) y (0, 1, 0) z (0, 0, 1) at (0, 0, 0)
component "Inside" placed x (1, 0, 0) y (0, 1, 0) z (0, 0, 1) at (0, 0, 0)
component "Copper Touch Pad" placed x (1, 0, 0) y (0, 1, 0) z (0, 0, 1) at (0, 0, 0)
component "Touch Test Block" placed x (1, 0, 0) y (0, 1, 0) z (0, 0, 1) at (0, 0, 0)
component "Inside w/ Touch and Ring" placed x (1, 0, 0) y (0, 1, 0) z (0, 0, 1) at (0, 0, 0)
component "Copper Touch Pad w/ Ring" placed x (1, 0, 0) y (0, 1, 0) z (0, 0, 1) at (0, 0, 0)
component "Inside w/ Touch and Ring" placed x (1, 0, 0) y (0, 1, 0) z (0, 0, 1) at (0, 0, 0)
component "Small Copper Touch Pad w/ Ring" placed x (1, 0, 0) y (0, 1, 0) z (0, 0, 1) at (0, 0, 0)
component "Inside w/ Small Touch" placed x (1, 0, 0) y (0, 1, 0) z (0, 0, 1) at (0, 0, 0)
component "Circular Touch" placed x (1, 0, 0) y (0, 1, 0) z (0, 0, 1) at (0, 0, 0)
component "Small Circular Touch" placed x (1, 0, 0) y (0, 1, 0) z (0, 0, 1) at (0, 0, 0)
component "Face" placed x (1, 0, 0) y (0, 1, 0) z (0, 0, 1) at (0, 0, 0)
hidden bodies 6 16 17
